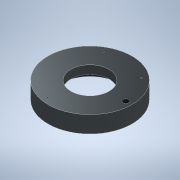
# Autodesk Inventor part: Корпус сальника 1
Saved by Autodesk Inventor 2021 (Build 250183000, 183)
## iProperties
Created: 2020-11-05
Part Number: Корпус сальника 1
Material: Чугун, серый
Document SubType Name: Modeling
Designer: Тимоха
Density: 7.15 g/cm^3
Appearance: Чугун серый
Mass: 1505.16 g
Surface Area: 407.904 cm^2
Volume: 210.512 cm^3
Author: Тимоха
Autodesk Inventor part; units mm, degrees
ref_plane "YZ Plane" through (0, 0, 0) normal (1, 0, 0) x (0, 1, 0)
ref_plane "XZ Plane" through (0, 0, 0) normal (0, 1, 0) x (-1, 0, 0)
ref_plane "XY Plane" through (0, 0, 0) normal (0, 0, 1) x (1, 0, 0)
sketch "Эскиз1" plane through (0, 0, 0) normal (0, 0, 1) x (1, 0, 0)
  line L0 (0, 0) -> (0, 20)
  line L1 (0, 0) -> (0, 24)
  line L2 (0, 0) -> (0, 30)
  line L3 (0, 30) -> (-75, 30)
  line L4 (-75, 30) -> (-75, 0)
  line L5 (-75, 0) -> (-51, 0)
  line L6 (-51, 0) -> (-51, 15)
  line L7 (-51, 15) -> (-34, 15)
  line L8 (-34, 15) -> (-34, 30)
  line L9 (-54, 27) -> (-39, 27)
  line L10 (-39, 27) -> (-39, 18)
  line L11 (-39, 18) -> (-54, 18)
  line L12 (-54, 18) -> (-54, 27)
  dimension "d20" = 30
  dimension "d21" = 75
  dimension "d22" = 24
  dimension "d23" = 15
  dimension "d24" = 17
  constraints: 26 end point, 6 perpendicular, 3 point on line, 2 horizontal, 2 parallel, 1 vertical
  measures "d20" distance of L0.start L2.end
  measures "d21" distance of L2.end L3.end
  measures "d22" distance of L4.end L5.end
  measures "d23" distance of L5.end L6.end
  measures "d24" distance of L6.end L7.end
revolve "Вращение1" add sketch "Эскиз1" angle 360 about axis through (0, 0, 0) along (0, 1, 0)
sketch "Эскиз2" plane through (0, 30, 0) normal (0, 1, 0) x (1, 0, 0)
  circle A0 centre (0, 0) radius 32 projected
  circle A1 centre (0, 0) radius 69 projected
  line L0 (0, 0) -> (41.7812, 49.7929)
  line L1 (0, 0) -> (65, 0) construction
  circle A2 centre (41.7812, 49.7929) radius 1.5
  line L2 (0, 0) -> (-32.5, 56.2917)
  line L3 (0, 0) -> (65, 0) construction
  circle A3 centre (-32.5, 56.2917) radius 1.5
  line L4 (0, 0) -> (-11.2871, -64.0125)
  line L5 (0, 0) -> (65, 0) construction
  circle A4 centre (-11.2871, -64.0125) radius 1.5
  dimension "d8" = 65
  dimension "d9" = 50
  dimension "d10" = 3
  dimension "d11" = 65
  dimension "d12" = 120
  dimension "d13" = 3
  dimension "d14" = 65
  dimension "d15" = 100
  dimension "d16" = 3
  constraints: 12 end point, 3 centre point, 3 coincident, 3 equal length, 3 horizontal, 1 point on line
  measures "d8" distance of L0.start L0.end
  measures "d9" angle of L1 L0
  measures "d10" diameter of A2
  measures "d11" distance of L0.start L2.end
  measures "d12" angle of L3 L2
  measures "d13" diameter of A3
  measures "d14" distance of L0.start L4.end
  measures "d15" angle of L4 L5
  measures "d16" diameter of A4
extrude "Выдавливание1" cut sketch "Эскиз2" against normal through all contours A2 | A3 | A4
sketch "Эскиз3" plane through (0, 0, 0) normal (0, 1, 0) x (-1, 0, 0)
  circle A0 centre (11.2871, 64.0125) radius 1.5 projected
  circle A1 centre (-41.7812, -49.7929) radius 1.5 projected
  circle A2 centre (32.5, -56.2917) radius 1.5 projected
  circle A3 centre (0, 0) radius 75 projected
  circle A4 centre (0, 0) radius 34 projected
  circle A5 centre (-64, 0) radius 5
  constraints: 1 centre point
extrude "Выдавливание2" cut sketch "Эскиз3" along normal through all contours A5
sketch "Эскиз4" plane through (0, 0, 0) normal (0, 1, 0) x (-1, 0, 0)
  circle A0 centre (-64, 0) radius 5 projected
  circle A1 centre (-64, 0) radius 6
  point P0 (0, 0)
  dimension "d27" = 12
  constraints: 1 centre point, 1 coincident
  measures "d27" diameter of A1
extrude "Выдавливание3" cut sketch "Эскиз4" along normal blind 1
